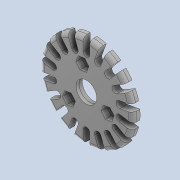
# Autodesk Inventor part: PartB
Saved by Autodesk Inventor 2020.4 (Build 244396000, 396)
## iProperties
Created: 2020-05-03
Part Number: PartB
Material: ABS Plastic
Document SubType Name: Modeling
Designer: Acer
Density: 1.06 g/cm^3
Appearance: Smooth - White
Author: Acer
Autodesk Inventor part; units mm, degrees
ref_plane "YZ Plane" through (0, 0, 0) normal (1, 0, 0) x (0, 1, 0)
ref_plane "XZ Plane" through (0, 0, 0) normal (0, 1, 0) x (-1, 0, 0)
ref_plane "XY Plane" through (0, 0, 0) normal (0, 0, 1) x (1, 0, 0)
sketch "Sketch1" plane through (0, 0, 0) normal (0, 0, 1) x (1, 0, 0)
  circle A0 centre (0, 0) radius 22.5
  dimension "d0" = 45
  constraints: 1 centre point, 1 coincident
  measures "d0" diameter of A0
extrude "PartB Base" add sketch "Sketch1" along normal blind 3.5
sketch "Sketch2" plane through (0, 0, 3.5) normal (0, 0, 1) x (1, 0, 0)
  line L0 (0, 22.95) -> (0, 16.25) construction
  line L1 (-1.6, 22.95) -> (-1.6, 16.25)
  line L2 (1.6, 16.25) -> (1.6, 22.95)
  arc A0 (1.6, 22.95) -> (-1.6, 22.95) centre (0, 22.95) ccw
  arc A1 (-1.6, 16.25) -> (1.6, 16.25) centre (0, 16.25) ccw
  arc A2 (-6.3459, 22.1132) -> (-9.3529, 21.0187) centre (-7.8494, 21.5659) ccw
  line L3 (-7.8494, 21.5659) -> (-5.5578, 15.27) construction
  line L4 (-4.0543, 15.8172) -> (-6.3459, 22.1132)
  arc A3 (-7.0613, 14.7228) -> (-4.0543, 15.8172) centre (-5.5578, 15.27) ccw
  line L5 (-9.3529, 21.0187) -> (-7.0613, 14.7228)
  arc A4 (-13.5263, 18.6092) -> (-15.9776, 16.5523) centre (-14.752, 17.5807) ccw
  line L6 (-14.752, 17.5807) -> (-10.4453, 12.4482) construction
  line L7 (-9.2196, 13.4767) -> (-13.5263, 18.6092)
  arc A5 (-11.671, 11.4198) -> (-9.2196, 13.4767) centre (-10.4453, 12.4482) ccw
  line L8 (-15.9776, 16.5523) -> (-11.671, 11.4198)
  arc A6 (-19.0753, 12.8606) -> (-20.6753, 10.0894) centre (-19.8753, 11.475) ccw
  line L9 (-19.8753, 11.475) -> (-14.0729, 8.125) construction
  line L10 (-13.2729, 9.5106) -> (-19.0753, 12.8606)
  arc A7 (-14.8729, 6.7394) -> (-13.2729, 9.5106) centre (-14.0729, 8.125) ccw
  line L11 (-20.6753, 10.0894) -> (-14.8729, 6.7394)
  arc A8 (-22.3235, 5.5609) -> (-22.8792, 2.4095) centre (-22.6013, 3.9852) ccw
  line L12 (-22.6013, 3.9852) -> (-16.0031, 2.8218) construction
  line L13 (-15.7253, 4.3975) -> (-22.3235, 5.5609)
  arc A9 (-16.281, 1.2461) -> (-15.7253, 4.3975) centre (-16.0031, 2.8218) ccw
  line L14 (-22.8792, 2.4095) -> (-16.281, 1.2461)
  arc A10 (-22.8792, -2.4095) -> (-22.3235, -5.5609) centre (-22.6013, -3.9852) ccw
  line L15 (-22.6013, -3.9852) -> (-16.0031, -2.8218) construction
  line L16 (-16.281, -1.2461) -> (-22.8792, -2.4095)
  arc A11 (-15.7253, -4.3975) -> (-16.281, -1.2461) centre (-16.0031, -2.8218) ccw
  line L17 (-22.3235, -5.5609) -> (-15.7253, -4.3975)
  arc A12 (-20.6753, -10.0894) -> (-19.0753, -12.8606) centre (-19.8753, -11.475) ccw
  line L18 (-19.8753, -11.475) -> (-14.0729, -8.125) construction
  line L19 (-14.8729, -6.7394) -> (-20.6753, -10.0894)
  arc A13 (-13.2729, -9.5106) -> (-14.8729, -6.7394) centre (-14.0729, -8.125) ccw
  line L20 (-19.0753, -12.8606) -> (-13.2729, -9.5106)
  arc A14 (-15.9776, -16.5523) -> (-13.5263, -18.6092) centre (-14.752, -17.5807) ccw
  line L21 (-14.752, -17.5807) -> (-10.4453, -12.4482) construction
  line L22 (-11.671, -11.4198) -> (-15.9776, -16.5523)
  arc A15 (-9.2196, -13.4767) -> (-11.671, -11.4198) centre (-10.4453, -12.4482) ccw
  line L23 (-13.5263, -18.6092) -> (-9.2196, -13.4767)
  arc A16 (-9.3529, -21.0187) -> (-6.3459, -22.1132) centre (-7.8494, -21.5659) ccw
  line L24 (-7.8494, -21.5659) -> (-5.5578, -15.27) construction
  line L25 (-7.0613, -14.7228) -> (-9.3529, -21.0187)
  arc A17 (-4.0543, -15.8172) -> (-7.0613, -14.7228) centre (-5.5578, -15.27) ccw
  line L26 (-6.3459, -22.1132) -> (-4.0543, -15.8172)
  arc A18 (-1.6, -22.95) -> (1.6, -22.95) centre (0, -22.95) ccw
  line L27 (0, -22.95) -> (0, -16.25) construction
  line L28 (-1.6, -16.25) -> (-1.6, -22.95)
  arc A19 (1.6, -16.25) -> (-1.6, -16.25) centre (0, -16.25) ccw
  line L29 (1.6, -22.95) -> (1.6, -16.25)
  arc A20 (6.3459, -22.1132) -> (9.3529, -21.0187) centre (7.8494, -21.5659) ccw
  line L30 (7.8494, -21.5659) -> (5.5578, -15.27) construction
  line L31 (4.0543, -15.8172) -> (6.3459, -22.1132)
  arc A21 (7.0613, -14.7228) -> (4.0543, -15.8172) centre (5.5578, -15.27) ccw
  line L32 (9.3529, -21.0187) -> (7.0613, -14.7228)
  arc A22 (13.5263, -18.6092) -> (15.9776, -16.5523) centre (14.752, -17.5807) ccw
  line L33 (14.752, -17.5807) -> (10.4453, -12.4482) construction
  line L34 (9.2196, -13.4767) -> (13.5263, -18.6092)
  arc A23 (11.671, -11.4198) -> (9.2196, -13.4767) centre (10.4453, -12.4482) ccw
  line L35 (15.9776, -16.5523) -> (11.671, -11.4198)
  arc A24 (19.0753, -12.8606) -> (20.6753, -10.0894) centre (19.8753, -11.475) ccw
  line L36 (19.8753, -11.475) -> (14.0729, -8.125) construction
  line L37 (13.2729, -9.5106) -> (19.0753, -12.8606)
  arc A25 (14.8729, -6.7394) -> (13.2729, -9.5106) centre (14.0729, -8.125) ccw
  line L38 (20.6753, -10.0894) -> (14.8729, -6.7394)
  arc A26 (22.3235, -5.5609) -> (22.8792, -2.4095) centre (22.6013, -3.9852) ccw
  line L39 (22.6013, -3.9852) -> (16.0031, -2.8218) construction
  line L40 (15.7253, -4.3975) -> (22.3235, -5.5609)
  arc A27 (16.281, -1.2461) -> (15.7253, -4.3975) centre (16.0031, -2.8218) ccw
  line L41 (22.8792, -2.4095) -> (16.281, -1.2461)
  arc A28 (22.8792, 2.4095) -> (22.3235, 5.5609) centre (22.6013, 3.9852) ccw
  line L42 (22.6013, 3.9852) -> (16.0031, 2.8218) construction
  line L43 (16.281, 1.2461) -> (22.8792, 2.4095)
  arc A29 (15.7253, 4.3975) -> (16.281, 1.2461) centre (16.0031, 2.8218) ccw
  line L44 (22.3235, 5.5609) -> (15.7253, 4.3975)
  arc A30 (20.6753, 10.0894) -> (19.0753, 12.8606) centre (19.8753, 11.475) ccw
  line L45 (19.8753, 11.475) -> (14.0729, 8.125) construction
  line L46 (14.8729, 6.7394) -> (20.6753, 10.0894)
  arc A31 (13.2729, 9.5106) -> (14.8729, 6.7394) centre (14.0729, 8.125) ccw
  line L47 (19.0753, 12.8606) -> (13.2729, 9.5106)
  arc A32 (15.9776, 16.5523) -> (13.5263, 18.6092) centre (14.752, 17.5807) ccw
  line L48 (14.752, 17.5807) -> (10.4453, 12.4482) construction
  line L49 (11.671, 11.4198) -> (15.9776, 16.5523)
  arc A33 (9.2196, 13.4767) -> (11.671, 11.4198) centre (10.4453, 12.4482) ccw
  line L50 (13.5263, 18.6092) -> (9.2196, 13.4767)
  arc A34 (9.3529, 21.0187) -> (6.3459, 22.1132) centre (7.8494, 21.5659) ccw
  line L51 (7.8494, 21.5659) -> (5.5578, 15.27) construction
  line L52 (7.0613, 14.7228) -> (9.3529, 21.0187)
  arc A35 (4.0543, 15.8172) -> (7.0613, 14.7228) centre (5.5578, 15.27) ccw
  line L53 (6.3459, 22.1132) -> (4.0543, 15.8172)
  point P0 (0, 0)
  point P1 (0, 19.6)
  dimension "d3" = 6.7
  dimension "d4" = 3.2
  dimension "d5" = 0
  dimension "d6" = 19.6
  dimension "d9" = 360
  constraints: 144 end point, 72 point on circle, 36 centre point, 4 tangent, 1 midpoint, 1 parallel, 1 vertical, 199 other
  measures "d3" distance of L0.start L0.end
  measures "d4" diameter of A1
  measures "d5" horizontal distance of point (0, 0) L0.end
  measures "d6" distance of point (0, 0) point (0, 19.6)
extrude "Roller Entrance" cut sketch "Sketch2" against normal up to surface (3.5 mm away)
sketch "Sketch3" plane through (0, 0, 0) normal (0, 0, -1) x (-1, 0, 0)
  point P0 (0, 0)
hole "Bearing Fit" at (0, 0, 0) direction (0, 0, 1) diameter 11 depth 2
sketch "Sketch4" plane through (0, 0, 3.5) normal (0, 0, 1) x (1, 0, 0)
  circle A0 centre (-1.9101, 10.833) radius 1.5
  circle A1 centre (-8.4266, -7.0707) radius 1.5
  circle A2 centre (10.3367, -3.7623) radius 1.5
  point P0 (0, 0)
  dimension "d20" = 3
  dimension "d21" = 1.9101
  dimension "d22" = 10.833
  dimension "d25" = 360
  constraints: 3 centre point, 7 other
  measures "d20" diameter of A0
  measures "d21" horizontal distance of point (0, 0) A0.centre
  measures "d22" vertical distance of A0.centre point (0, 0)
extrude "Threads Fit" cut sketch "Sketch4" against normal up to surface (3.5 mm away)
sketch "Sketch5" plane through (0, 0, 3.5) normal (0, 0, 1) x (1, 0, 0)
  circle A0 centre (-1.9101, 10.833) radius 1.5 projected
  circle A1 centre (10.3367, -3.7623) radius 1.5 projected
  circle A2 centre (-8.4266, -7.0707) radius 1.5 projected
  line L0 (0, 0) -> (-1.9101, 10.833) construction
  circle A3 centre (10.3367, -3.7623) radius 1.5 projected
  line L1 (0, 0) -> (10.3367, -3.7623) construction
  line L2 (0, 0) -> (-8.4266, -7.0707) construction
  line L3 (-3.0001, 7.8382) -> (-5.0487, 10.2796)
  line L4 (-5.0487, 10.2796) -> (-3.9587, 13.2744)
  line L5 (-3.9587, 13.2744) -> (-0.8201, 13.8278)
  line L6 (-0.8201, 13.8278) -> (1.2284, 11.3864)
  line L7 (1.2284, 11.3864) -> (0.1384, 8.3916)
  line L8 (0.1384, 8.3916) -> (-3.0001, 7.8382)
  line L9 (8.2882, -1.3209) -> (11.4267, -0.7675)
  line L10 (11.4267, -0.7675) -> (13.4753, -3.2089)
  line L11 (13.4753, -3.2089) -> (12.3853, -6.2036)
  line L12 (12.3853, -6.2036) -> (9.2467, -6.7571)
  line L13 (9.2467, -6.7571) -> (7.1982, -4.3157)
  line L14 (7.1982, -4.3157) -> (8.2882, -1.3209)
  circle A4 centre (-8.4266, -7.0707) radius 1.5 projected
  line L15 (-5.288, -6.5173) -> (-6.378, -9.5121)
  line L16 (-6.378, -9.5121) -> (-9.5166, -10.0655)
  line L17 (-9.5166, -10.0655) -> (-11.5651, -7.6241)
  line L18 (-11.5651, -7.6241) -> (-10.4751, -4.6294)
  line L19 (-10.4751, -4.6294) -> (-7.3366, -4.0759)
  line L20 (-7.3366, -4.0759) -> (-5.288, -6.5173)
  point P0 (-1.4309, 8.1149)
  point P1 (7.7432, -2.8183)
  point P2 (-6.3123, -5.2966)
  dimension "d29" = 2.76
  dimension "d30" = 2.76
  dimension "d31" = 2.76
  constraints: 42 end point, 4 coincident, 3 midpoint, 3 point on line, 39 other
  measures "d29" distance from line of L20 L2.end
  measures "d30" distance from line of L14 L1.end
  measures "d31" distance from line of L8 L0.end
extrude "Extrusion4" cut sketch "Sketch5" against normal blind 2.75
sketch "Sketch6" plane through (0, 0, 3.5) normal (0, 0, 1) x (1, 0, 0)
  point P0 (0, 0)
hole "Thread Fit" at (0, 0, 3.5) direction (0, 0, -1) diameter 10 depth 1.5
fillet "Ground Round" radius 2 18 edges at (-11.25, 19.4856, 3.5) (-3.9071, 22.1582, 3.5) (3.9071, 22.1582, 3.5) (11.25, 19.4856, 3.5) (17.236, 14.4627, 3.5) (21.1431, 7.6955, 3.5) (22.5, 0, 3.5) (21.1431, -7.6955, 3.5) (17.236, -14.4627, 3.5) (11.25, -19.4856, 3.5) (3.9071, -22.1582, 3.5) (-3.9071, -22.1582, 3.5) (-11.25, -19.4856, 3.5) (-17.236, -14.4627, 3.5) (-21.1431, -7.6955, 3.5) (-22.5, 0, 3.5) (-17.236, 14.4627, 3.5) (-21.1431, 7.6955, 3.5)
body "Solid1"
